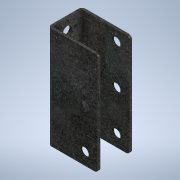
# Autodesk Inventor part: основа
Saved by Autodesk Inventor 2020.1 (Build 241239000, 239)
## iProperties
Created: 2021-08-17
Part Number: основа
Material: Сталь
Document SubType Name: Modeling
Designer: Ni3na
Density: 7.85 g/cm^3
Appearance: Листовая
Author: Ni3na
Autodesk Inventor part; units mm, degrees
ref_plane "YZ Plane" through (0, 0, 0) normal (1, 0, 0) x (0, 1, 0)
ref_plane "XZ Plane" through (0, 0, 0) normal (0, 1, 0) x (-1, 0, 0)
ref_plane "XY Plane" through (0, 0, 0) normal (0, 0, 1) x (1, 0, 0)
sketch "Эскиз1" plane through (0, 0, 0) normal (0, 0, 1) x (1, 0, 0)
  line L0 (-20.241, 29.4578) -> (24.759, 29.4578)
  line L1 (24.759, 29.4578) -> (24.759, -60.5422)
  line L2 (24.759, -60.5422) -> (-20.241, -60.5422)
  line L3 (-20.241, -60.5422) -> (-20.241, 29.4578)
  point P0 (0, 0)
  dimension "d0" = 90
  dimension "d1" = 45
  constraints: 8 end point, 2 parallel, 1 horizontal, 1 perpendicular
  measures "d0" distance of L1.end L0.end
  measures "d1" distance of L1.end L2.end
extrude "Выдавливание1" add sketch "Эскиз1" along normal blind 2
sketch "Эскиз2" plane through (0, 0, 2) normal (0, 0, 1) x (1, 0, 0)
  line L0 (-20.241, 29.4578) -> (-20.241, -60.5422) projected
  line L1 (-20.241, -60.5422) -> (24.759, -60.5422) projected
  line L2 (-20.241, 29.4578) -> (-18.241, 29.4578)
  line L3 (-18.241, 29.4578) -> (-18.241, -60.5422)
  line L4 (-18.241, -60.5422) -> (-20.241, -60.5422)
  line L5 (-20.241, -60.5422) -> (-20.241, 29.4578)
  point P0 (0, 0)
  dimension "d4" = 2
  constraints: 8 end point, 2 parallel, 1 horizontal, 1 perpendicular, 1 point on line
  measures "d4" distance of L3.end L0.end
extrude "Выдавливание2" add sketch "Эскиз2" along normal blind 28
sketch "Эскиз4" plane through (-20.241, 29.4578, 0) normal (0, 1, 0) x (1, 0, 0)
  line L0 (59.015, -17.4368) -> (44, -17.4368)
  line L1 (44, -17.4368) -> (44, 13.0776)
  line L2 (44, 13.0776) -> (59.015, 13.0776)
  line L3 (59.015, 13.0776) -> (59.015, -17.4368)
  line L4 (0, 0) -> (45, 0) projected
  point P0 (20.241, 0)
  point P1 (44, 0)
  point P2 (44, 0)
  point P3 (0, 0)
  dimension "d10" = 0
  dimension "d11" = 44
  constraints: 8 end point, 3 point on line, 2 parallel, 1 horizontal, 1 perpendicular
  measures "d10" distance of point (44, 0) point (44, 0)
  measures "d11" distance of L4.start point (44, 0)
extrude "Выдавливание4" cut sketch "Эскиз4" against normal blind 1000
sketch "Эскиз5" plane through (-18.241, -60.5422, 2) normal (1, 0, 0) x (0, 0, -1)
  line L0 (2, 0) -> (-28, 0) projected
  line L1 (0, 90) -> (-28, 90) projected
  line L2 (-28, 0) -> (-26, 0)
  line L3 (-26, 0) -> (-26, 90)
  line L4 (-26, 90) -> (-28, 90)
  line L5 (-28, 90) -> (-28, 0)
  point P0 (2, 60.5422)
  point P1 (-26, 0)
  dimension "d14" = 2
  constraints: 8 end point, 2 parallel, 1 horizontal, 1 perpendicular, 1 point on line
  measures "d14" distance of L3.end L1.end
extrude "Выдавливание5" add sketch "Эскиз5" along normal blind 42
sketch "Эскиз6" plane through (-18.241, -60.5422, 2) normal (1, 0, 0) x (0, 0, -1)
  circle A0 centre (-13, 80) radius 4
  line L0 (0, 90) -> (-26, 90) projected
  circle A1 centre (-13, 87) radius 1.5
  circle A2 centre (-20, 80) radius 1.5
  circle A3 centre (-13, 73) radius 1.5
  circle A4 centre (-6, 80) radius 1.5
  circle A5 centre (-13, 80) radius 7
  circle A6 centre (-13, 45) radius 4
  circle A7 centre (-20, 45) radius 1.5
  circle A8 centre (-13, 38) radius 1.5
  circle A9 centre (-6, 45) radius 1.5
  circle A10 centre (-13, 45) radius 7
  circle A11 centre (-13, 10) radius 4
  circle A12 centre (-20, 10) radius 1.5
  circle A13 centre (-13, 3) radius 1.5
  circle A14 centre (-6, 10) radius 1.5
  circle A15 centre (-13, 10) radius 7
  circle A16 centre (-13, 52) radius 1.5
  circle A17 centre (-13, 17) radius 1.5
  line L1 (2, 0) -> (-28, 0) projected
  line L2 (2, 90) -> (2, 0) projected
  point P0 (2, 60.5422)
  point P1 (-13, 90)
  point P2 (-13, 0)
  dimension "d17" = 8
  dimension "d19" = 0
  dimension "d21" = 14
  dimension "d22" = 3
  dimension "d23" = 3
  dimension "d24" = 3
  dimension "d25" = 3
  dimension "d26" = 0
  dimension "d27" = 0
  dimension "d28" = 7
  dimension "d29" = 7
  dimension "d30" = 0
  dimension "d31" = 7
  dimension "d32" = 0
  dimension "d33" = 7
  dimension "d34" = 8
  dimension "d35" = 14
  dimension "d36" = 3
  dimension "d37" = 3
  dimension "d38" = 3
  dimension "d39" = 0
  dimension "d40" = 0
  dimension "d41" = 7
  dimension "d42" = 7
  dimension "d43" = 0
  dimension "d44" = 7
  dimension "d45" = 0
  dimension "d46" = 7
  dimension "d47" = 8
  dimension "d48" = 14
  dimension "d49" = 3
  dimension "d50" = 3
  dimension "d51" = 3
  dimension "d52" = 0
  dimension "d53" = 0
  dimension "d54" = 7
  dimension "d55" = 7
  dimension "d56" = 0
  dimension "d57" = 7
  dimension "d58" = 0
  dimension "d59" = 7
  dimension "d60" = 3
  dimension "d61" = 3
  dimension "d65" = 17
  dimension "d67" = 10
  dimension "d68" = 21
  dimension "d69" = 15
  dimension "d70" = 15
  constraints: 18 centre point, 5 coincident, 2 midpoint
  measures "d17" diameter of A0
  measures "d19" horizontal distance of point (-13, 90) A0.centre
  measures "d21" diameter of A5
  measures "d22" diameter of A3
  measures "d23" diameter of A4
  measures "d24" diameter of A1
  measures "d25" diameter of A2
  measures "d26" vertical distance of A4.centre A0.centre
  measures "d27" horizontal distance of A1.centre A0.centre
  measures "d28" distance of A1.centre A0.centre
  measures "d29" distance of A4.centre A0.centre
  measures "d30" horizontal distance of A1.centre A3.centre
  measures "d31" distance of A3.centre A0.centre
  measures "d32" vertical distance of A0.centre A2.centre
  measures "d33" distance of A0.centre A2.centre
  measures "d34" diameter of A6
  measures "d35" diameter of A10
  measures "d36" diameter of A8
  measures "d37" diameter of A9
  measures "d38" diameter of A7
  measures "d39" vertical distance of A9.centre A6.centre
  measures "d40" horizontal distance of point (-13, 52) A6.centre
  measures "d41" distance of point (-13, 52) A6.centre
  measures "d42" distance of A9.centre A6.centre
  measures "d43" horizontal distance of point (-13, 52) A8.centre
  measures "d44" distance of A8.centre A6.centre
  measures "d45" vertical distance of A6.centre A7.centre
  measures "d46" distance of A6.centre A7.centre
  measures "d47" diameter of A11
  measures "d48" diameter of A15
  measures "d49" diameter of A13
  measures "d50" diameter of A14
  measures "d51" diameter of A12
  measures "d52" vertical distance of A14.centre A11.centre
  measures "d53" horizontal distance of point (-13, 17) A11.centre
  measures "d54" distance of point (-13, 17) A11.centre
  measures "d55" distance of A14.centre A11.centre
  measures "d56" horizontal distance of point (-13, 17) A13.centre
  measures "d57" distance of A13.centre A11.centre
  measures "d58" vertical distance of A11.centre A12.centre
  measures "d59" distance of A11.centre A12.centre
  measures "d60" diameter of A16
  measures "d61" diameter of A17
  measures "d65" distance of A3.centre point (-13, 90)
  measures "d67" distance of point (-13, 0) A11.centre
  measures "d68" distance of point (-13, 52) A3.centre
  measures "d69" distance from line of L2 A11.centre
  measures "d70" distance from line of L2 A6.centre
extrude "Выдавливание6" cut sketch "Эскиз6" against normal blind 5 contours A0 | A1 A5 | A5 A1 | A5 A2 | A2 A5 | A5 A4 | A4 A5 | A5 A3 | A3 A5 | A6 | A7 A10 | A10 A7 | A16 A10 | A10 A16 | A10 A8 | A8 A10 | A10 A9 | A9 A10 | A11 | A12 A15 | A15 A12 | A17 A15 | A15 A17 | A15 A13 | A13 A15 | A15 A14 | A14 A15
sketch "Эскиз7" plane through (0, 0, 30) normal (0, 0, 1) x (1, 0, 0)
  circle A0 centre (11.759, 19.4578) radius 4
  circle A1 centre (11.759, 19.4578) radius 7
  circle A2 centre (4.759, 19.4578) radius 1.5
  circle A3 centre (11.759, 12.4578) radius 1.5
  circle A4 centre (18.759, 19.4578) radius 1.5
  circle A5 centre (11.759, 26.4578) radius 1.5
  line L0 (23.759, 29.4578) -> (23.759, -60.5422) projected
  line L1 (23.759, 29.4578) -> (-18.241, 29.4578) projected
  circle A6 centre (11.759, -15.5422) radius 4
  circle A7 centre (11.759, -15.5422) radius 7
  circle A8 centre (11.759, -22.5422) radius 1.5
  circle A9 centre (18.759, -15.5422) radius 1.5
  circle A10 centre (11.7213, -8.5423) radius 1.5
  circle A11 centre (11.759, -50.5422) radius 4
  circle A12 centre (11.759, -50.5422) radius 7
  circle A13 centre (11.759, -57.5422) radius 1.5
  circle A14 centre (18.759, -50.5422) radius 1.5
  circle A15 centre (11.759, -43.5422) radius 1.5
  line L2 (-20.241, -60.5422) -> (23.759, -60.5422) projected
  circle A16 centre (4.759, -15.5422) radius 1.5
  circle A17 centre (4.759, -50.5422) radius 1.5
  point P0 (0, 0)
  point P1 (23.759, 19.4578)
  point P2 (11.759, 29.4578)
  dimension "d73" = 8
  dimension "d74" = 14
  dimension "d75" = 3
  dimension "d76" = 3
  dimension "d77" = 3
  dimension "d78" = 3
  dimension "d80" = 0
  dimension "d81" = 12
  dimension "d82" = 0
  dimension "d83" = 0
  dimension "d84" = 7
  dimension "d85" = 0
  dimension "d86" = 7
  dimension "d87" = 7
  dimension "d88" = 8
  dimension "d89" = 14
  dimension "d91" = 3
  dimension "d92" = 3
  dimension "d93" = 3
  dimension "d94" = 0
  dimension "d95" = 7
  dimension "d96" = 0
  dimension "d97" = 7
  dimension "d98" = 7
  dimension "d99" = 8
  dimension "d100" = 14
  dimension "d102" = 3
  dimension "d103" = 3
  dimension "d104" = 3
  dimension "d105" = 0
  dimension "d106" = 7
  dimension "d107" = 0
  dimension "d108" = 7
  dimension "d109" = 7
  dimension "d110" = 0
  dimension "d111" = 0
  dimension "d112" = 0
  dimension "d114" = 35
  dimension "d115" = 35
  dimension "d116" = 3
  dimension "d117" = 3
  dimension "d118" = 3
  constraints: 18 centre point, 9 point on circle, 4 coincident, 2 point on line
  measures "d73" diameter of A0
  measures "d74" diameter of A1
  measures "d75" diameter of A2
  measures "d76" diameter of A3
  measures "d77" diameter of A4
  measures "d78" diameter of A5
  measures "d80" vertical distance of point (23.759, 19.458) A0.centre
  measures "d81" distance of point (23.759, 29.458) point (11.759, 29.458)
  measures "d82" horizontal distance of point (11.759, 29.458) A0.centre
  measures "d83" vertical distance of A4.centre A0.centre
  measures "d84" distance of A0.centre A4.centre
  measures "d85" horizontal distance of A0.centre A3.centre
  measures "d86" distance of A0.centre A3.centre
  measures "d87" distance of A5.centre A0.centre
  measures "d88" diameter of A6
  measures "d89" diameter of A7
  measures "d91" diameter of A8
  measures "d92" diameter of A9
  measures "d93" diameter of A10
  measures "d94" vertical distance of A9.centre A6.centre
  measures "d95" distance of A6.centre A9.centre
  measures "d96" horizontal distance of A6.centre A8.centre
  measures "d97" distance of A6.centre A8.centre
  measures "d98" distance of A10.centre A6.centre
  measures "d99" diameter of A11
  measures "d100" diameter of A12
  measures "d102" diameter of A13
  measures "d103" diameter of A14
  measures "d104" diameter of A15
  measures "d105" vertical distance of A14.centre A11.centre
  measures "d106" distance of A11.centre A14.centre
  measures "d107" horizontal distance of A11.centre A13.centre
  measures "d108" distance of A11.centre A13.centre
  measures "d109" distance of A15.centre A11.centre
  measures "d110" horizontal distance of A11.centre A15.centre
  measures "d111" horizontal distance of A6.centre A0.centre
  measures "d112" horizontal distance of A11.centre A6.centre
  measures "d114" distance of A6.centre A1.centre
  measures "d115" distance of A6.centre A11.centre
  measures "d116" distance of point (11.759, 29.458) A5.centre
  measures "d117" diameter of A16
  measures "d118" diameter of A17
extrude "Выдавливание7" cut sketch "Эскиз7" against normal blind 100 contours A0 | A1 A4 | A1 A4 | A5 A1 | A1 A5 | A3 A1 | A1 A3 | A2 A1 | A1 A2 | A6 | A7 A9 | A7 A9 | A10 A7 | A7 A10 | A8 A7 | A7 A8 | A16 A7 | A7 A16 | A11 | A12 A14 | A12 A14 | A15 A12 | A12 A15 | A13 A12 | A12 A13 | A17 A12 | A12 A17
sketch "Эскиз8" plane through (0, 0, 30) normal (0, 0, 1) x (1, 0, 0)
  circle A0 centre (18.259, -2.0422) radius 1.5
  circle A1 centre (18.259, -29.0422) radius 1.5
  line L0 (-20.241, 29.4578) -> (23.759, 29.4578) projected
  line L1 (23.759, 29.4578) -> (23.759, -60.5422) projected
  point P0 (0, 0)
  dimension "d121" = 3
  dimension "d122" = 3
  dimension "d123" = 31.5
  dimension "d124" = 5.5
  dimension "d125" = 0
  dimension "d126" = 27
  constraints: 2 centre point
  measures "d121" diameter of A0
  measures "d122" diameter of A1
  measures "d123" distance from line of A0.centre L0
  measures "d124" distance from line of L1 A0.centre
  measures "d125" horizontal distance of A0.centre A1.centre
  measures "d126" distance of A0.centre A1.centre
extrude "Выдавливание8" cut sketch "Эскиз8" against normal blind 100
fillet "Сопряжение1" radius 3 6 edges at (-20.241, -15.5422, 30) (23.759, 29.4578, 29) (23.759, 29.4578, 1) (23.759, -60.5422, 29) (23.759, -60.5422, 1) (-20.241, -15.5422, 0)
